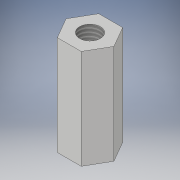
# Autodesk Inventor part: 12mm_Innengewinde
Saved by Autodesk Inventor 2017.3 (Build 213257000, 257)
## iProperties
Part Number: 12mm_Innengewinde
Material: Generisch
Document SubType Name: Modeling
Designer: Enno-LT
Density: 1 g/cm^3
Appearance: Vorgabe
Author: Enno-LT
Autodesk Inventor part; units mm, degrees
ref_plane "YZ Plane" through (0, 0, 0) normal (1, 0, 0) x (0, 1, 0)
ref_plane "XZ Plane" through (0, 0, 0) normal (0, 1, 0) x (-1, 0, 0)
ref_plane "XY Plane" through (0, 0, 0) normal (0, 0, 1) x (1, 0, 0)
sketch "Skizze1" plane through (0, 0, 0) normal (0, 0, 1) x (1, 0, 0)
  line L0 (-1.4434, 2.5) -> (1.4434, 2.5)
  line L1 (1.4434, 2.5) -> (2.8868, 0)
  line L2 (2.8868, 0) -> (1.4434, -2.5)
  line L3 (1.4434, -2.5) -> (-1.4434, -2.5)
  line L4 (-1.4434, -2.5) -> (-2.8868, 0)
  line L5 (-2.8868, 0) -> (-1.4434, 2.5)
  point P0 (0, 0)
  point P1 (0, 0)
  point P2 (0, 2.5)
  point P3 (0, -2.5)
  dimension "d3" = 120
  dimension "d4" = 120
  dimension "d5" = 120
  dimension "d6" = 5
  constraints: 12 end point, 2 equal length, 2 horizontal alignment, 2 midpoint, 2 vertical alignment, 1 coincident, 1 horizontal, 1 parallel
  measures "d3" angle of L5 L0
  measures "d4" angle of L1 L0
  measures "d5" angle of L2 L3
  measures "d6" distance between parallel lines of L3 L0
extrude "Extrusion1" add sketch "Skizze1" along normal blind 12
sketch "Skizze2" plane through (0, 0, 12) normal (0, 0, 1) x (1, 0, 0)
  point P0 (0, 0)
  point P1 (0, 0)
  constraints: 1 coincident
hole "Bohrung1" at (0, 0, 12) direction (0, 0, -1) diameter 2.5 end through all
thread "Gewinde1" size "M2.5x0.45" class "6H" standard "ANSI Metric M Profile" full length
